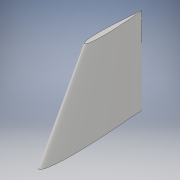
# Autodesk Inventor part: vTail_wing
Saved by Autodesk Inventor 2019 (Build 230136000, 136)
## iProperties
Created: 2019-04-06
Part Number: vTail_wing
Material: Generic_532
Document SubType Name: Modeling
Designer: albaa
Density: 0.03 g/cm^3
Appearance: Default(1)
Mass: 5.60064 g
Surface Area: 453 cm^2
Volume: 186.688 cm^3
Author: albaa
Autodesk Inventor part; units mm, degrees
ref_plane "YZ Plane" through (0, 0, 0) normal (1, 0, 0) x (0, 1, 0)
ref_plane "XY Plane" through (0, 0, 0) normal (0, 0, 1) x (1, 0, 0)
sketch "Sketch1" plane through (0, 0, 0) normal (0, 1, 0) x (-1, 0, 0)
  spline S0 degree 5 poles (0.1701, -180) (0.6947, -179.3517) (1.4348, -174.0248) (1.6083, -156.5866) (3.3071, -153.0966) (4.1507, -134.1897) (5.3126, -122.4813) (6.166, -107.9136) (6.9493, -94.942) (7.5263, -82.1159) (7.9311, -70.1269) (8.1293, -58.8226) (8.1283, -48.3717) (7.9095, -38.8052) (7.5104, -30.2149) (6.891, -22.6268) (6.1687, -16.1391) (5.2107, -10.6988) (4.2865, -6.4152) (3.037, -3.0393) (1.8987, -0.7658) (0, 0.6342) (-1.8987, -0.7658) (-3.037, -3.0393) (-4.2865, -6.4152) (-5.2107, -10.6988) (-6.1687, -16.1391) (-6.891, -22.6268) (-7.5104, -30.2149) (-7.9094, -38.8052) (-8.1285, -48.3717) (-8.1288, -58.8226) (-7.9324, -70.127) (-7.5229, -82.1156) (-6.9583, -94.9427) (-6.1429, -107.9117) (-5.3707, -122.4859) (-4.0067, -134.2547) (-3.6699, -151.1667) (-1.3169, -156.2697) (-1.7714, -172.6555) (-0.7605, -179.4651) (-0.1324, -180.3738) (0.1701, -180) knots 0 0 0 0 0 0 0.040547 0.067415 0.10082 0.133863 0.166426 0.19839 0.229632 0.260026 0.289442 0.317745 0.344792 0.37043 0.394489 0.416782 0.437092 0.455184 0.470925 0.484705 0.497442 0.51018 0.52396 0.539701 0.557793 0.578103 0.600395 0.624455 0.650093 0.67714 0.705443 0.734859 0.765253 0.796495 0.828459 0.861022 0.894065 0.92747 0.955361 0.97662 1 1 1 1 1 1
  point P0 (0, 0)
  point P1 (0, 0)
  point P2 (1.3703, -0.6148)
  point P3 (2.6641, -2.455)
  point P4 (3.8685, -5.508)
  point P5 (4.9649, -9.7529)
  point P6 (5.9311, -15.1608)
  point P7 (6.7438, -21.6947)
  point P8 (7.381, -29.31)
  point P9 (7.8245, -37.9547)
  point P10 (8.0617, -47.5697)
  point P11 (8.0869, -58.0893)
  point P12 (7.9013, -69.4417)
  point P13 (7.5127, -81.5493)
  point P14 (6.9337, -94.3295)
  point P15 (6.1793, -107.6948)
  point P16 (5.2649, -121.5541)
  point P17 (4.2028, -135.8126)
  point P18 (3.0005, -150.373)
  point P19 (0, 0)
  point P20 (-1.3703, -0.6148)
  point P21 (-2.6641, -2.455)
  point P22 (-3.8685, -5.508)
  point P23 (-4.9649, -9.7529)
  point P24 (-5.9311, -15.1608)
  point P25 (-6.7438, -21.6947)
  point P26 (-7.381, -29.31)
  point P27 (-7.8245, -37.9547)
  point P28 (-8.0617, -47.5697)
  point P29 (-8.0869, -58.0893)
  point P30 (-7.9013, -69.4417)
  point P31 (-7.5127, -81.5493)
  point P32 (-6.9337, -94.3295)
  point P33 (-6.1793, -107.6948)
  point P34 (-5.2649, -121.5541)
  point P35 (-4.2028, -135.8126)
  point P36 (-3.0005, -150.373)
  point P37 (-1.6586, -165.1357)
  point P38 (-0.1701, -180)
  point P39 (6.9337, -94.3295)
  constraints: 1 coincident, 40 other
ref_plane "Work Plane1" through (0, 150, 0) normal (0, 1, 0) x (-1, 0, 0)
sketch "Sketch2" plane through (0, 150, 0) normal (0, 1, 0) x (-1, 0, 0)
  spline S0 degree 5 poles (0.0945, -180) (0.386, -179.6399) (0.7971, -176.6805) (0.8935, -166.9926) (1.8373, -165.0537) (2.3059, -154.5498) (2.9516, -148.0451) (3.4253, -139.9521) (3.8613, -132.7453) (4.1801, -125.6205) (4.4087, -118.9582) (4.5111, -112.6816) (4.5258, -106.8685) (4.3749, -101.5673) (4.2078, -96.7698) (3.7661, -92.5991) (3.5303, -88.9187) (2.7297, -85.9953) (2.6036, -83.3827) (1.2802, -81.7) (1.5111, -79.9687) (-1.5111, -79.9687) (-1.2802, -81.7) (-2.6036, -83.3827) (-2.7297, -85.9953) (-3.5303, -88.9187) (-3.7661, -92.5991) (-4.2078, -96.7698) (-4.3749, -101.5673) (-4.5259, -106.8685) (-4.5109, -112.6816) (-4.4095, -118.9583) (-4.1781, -125.6203) (-3.8663, -132.7457) (-3.4124, -139.9511) (-2.9839, -148.0477) (-2.2259, -154.586) (-2.0388, -163.9815) (-0.7316, -166.8165) (-0.9841, -175.9197) (-0.4225, -179.7029) (-0.0736, -180.2077) (0.0945, -180) knots 0 0 0 0 0 0 0.040832 0.067889 0.101528 0.134803 0.167596 0.199784 0.231245 0.261853 0.291476 0.319978 0.347215 0.373032 0.397261 0.419711 0.440163 0.458382 0.474993 0.490114 0.504735 0.519856 0.536467 0.554686 0.575138 0.597588 0.621817 0.647634 0.674871 0.703373 0.732996 0.763604 0.795065 0.827253 0.860046 0.893321 0.92696 0.955047 0.976456 1 1 1 1 1 1
  point P0 (0, -80)
  point P1 (0.7613, -80.3416)
  point P2 (1.4801, -81.3639)
  point P3 (2.1492, -83.06)
  point P4 (2.7583, -85.4183)
  point P5 (3.2951, -88.4227)
  point P6 (3.7466, -92.0526)
  point P7 (4.1006, -96.2834)
  point P8 (4.3469, -101.0859)
  point P9 (4.4787, -106.4276)
  point P10 (4.4927, -112.2718)
  point P11 (4.3896, -118.5787)
  point P12 (4.1737, -125.3052)
  point P13 (3.852, -132.4053)
  point P14 (3.433, -139.8305)
  point P15 (2.9249, -147.5301)
  point P16 (2.3349, -155.4515)
  point P17 (1.6669, -163.5405)
  point P18 (0, -80)
  point P19 (-0.7613, -80.3416)
  point P20 (-1.4801, -81.3639)
  point P21 (-2.1492, -83.06)
  point P22 (-2.7583, -85.4183)
  point P23 (-3.2951, -88.4227)
  point P24 (-3.7466, -92.0526)
  point P25 (-4.1006, -96.2834)
  point P26 (-4.3469, -101.0859)
  point P27 (-4.4787, -106.4276)
  point P28 (-4.4927, -112.2718)
  point P29 (-4.3896, -118.5787)
  point P30 (-4.1737, -125.3052)
  point P31 (-3.852, -132.4053)
  point P32 (-3.433, -139.8305)
  point P33 (-2.9249, -147.5301)
  point P34 (-2.3349, -155.4515)
  point P35 (-1.6669, -163.5405)
  point P36 (-0.9214, -171.7421)
  point P37 (-0.0945, -180)
  point P38 (0, -80)
  constraints: 1 coincident, 38 other
loft "Loft1" add profiles "Sketch1", "Sketch2"
body "Solid1"
